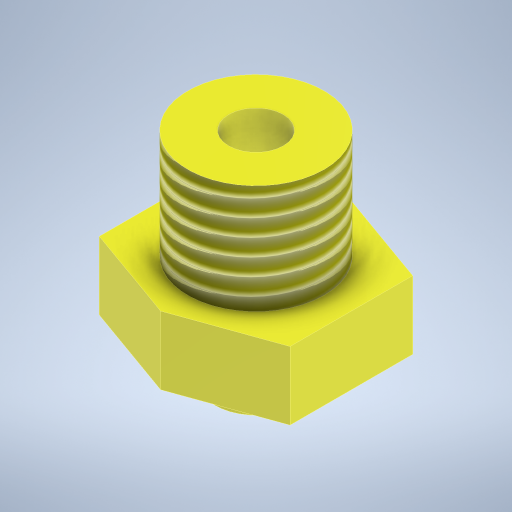
# Autodesk Inventor part: 1-HUDSON-8-30-TDR HAND PUMP BODY BOTTOM INLET
Saved by Autodesk Inventor 2024.2 (Build 282272000, 272)
## iProperties
Created: 2024-11-02
Part Number: 1-HUDSON-8-30-TDR HAND PUMP BODY BOTTOM INLET
Material: Genérico
Document SubType Name: Modeling
Designer: brene
Density: 1 g/cm^3
Appearance: Amarillo
Author: brene
Autodesk Inventor part; units mm, degrees
ref_plane "YZ Plane" through (0, 0, 0) normal (1, 0, 0) x (0, 1, 0)
ref_plane "XZ Plane" through (0, 0, 0) normal (0, 1, 0) x (-1, 0, 0)
ref_plane "XY Plane" through (0, 0, 0) normal (0, 0, 1) x (1, 0, 0)
sketch "Boceto1" plane through (0, 0, 0) normal (0, 0, 1) x (1, 0, 0)
  line L0 (0, 21.3006) -> (0, 0)
  line L1 (0, 15.4538) -> (5, 15.4538)
  line L2 (5, 15.4538) -> (5, 7.4538)
  line L3 (5, 7.4538) -> (0, 7.4538)
  line L4 (7, 7.4538) -> (5, 7.4538)
  line L5 (7, 7.4538) -> (7, 2.4538)
  line L6 (7, 2.4538) -> (0, 2.4538)
  line L7 (3, 2.4538) -> (3, 0.9538)
  line L8 (2, 15.4538) -> (2, -0.5462)
  line L9 (3, -0.5462) -> (2, -0.5462)
  line L10 (0, 0.6254) -> (0, -1.387)
  line L11 (3, -0.5462) -> (3, -0.5462)
  arc A0 (6, 2.4538) -> (3, -0.5462) centre (6, -0.5462) ccw
  line L12 (3, 0.9538) -> (3, -0.5462)
  point P0 (2, 2.4538)
  point P1 (2, 7.4538)
  dimension "d0" = 10
  dimension "d1" = 4
  dimension "d2" = 14
  dimension "d4" = 5
  dimension "d6" = 8
  dimension "d9" = 15.4538
  dimension "d10" = 13.8468
  dimension "d11" = 1.8283
  dimension "d12" = 3.8408
  dimension "d16" = 3
  dimension "d17" = 1
  dimension "d18" = 4
  dimension "d19" = 0.5462
  dimension "d20" = 6
  dimension "d21" = 1
  constraints: 26 end point, 8 point on line, 5 vertical, 3 perpendicular, 2 horizontal, 2 point on circle, 1 centre point, 1 collinear, 1 tangent
  measures "d0" diameter of L2 L0
  measures "d1" diameter of L8 L0
  measures "d2" diameter of L5 L0
  measures "d4" distance of L4.start L5.end
  measures "d6" distance of L1.end L2.end
  measures "d9" distance from line of L0.end L1
  measures "d10" distance from line of L0.start L4
  measures "d11" distance from line of L10.start L6
  measures "d12" distance from line of L10.end L6
  measures "d16" distance of L9.start L7.start
  measures "d17" distance of L9.start L8.end
  measures "d18" diameter of L8.end L10
  measures "d19" distance from line of L9 L0.end
  measures "d20" diameter of L7 L0
  measures "d21" distance of L5.end A0.start
revolve "Revolución1" add sketch "Boceto1" angle 360 about axis through (0, 21.3006, 0) along (0, -1, 0) contours L1 L2 L3 L8 | L3 L4 L5 L6 L8 | L6 L7 L12 L9 L8
revolve "Revolución2" add sketch "Boceto1" angle 360 about axis through (0, 0.6254, 0) along (0, -1, 0) contours L6 A0 L12 L7
sketch "Boceto2" plane through (0, 7.4538, 0) normal (0, 1, 0) x (1, 0, 0)
  line L0 (0, 11.3393) -> (0, -11.3393) construction
  line L1 (-23.3185, 0) -> (23.3185, 0) construction
  line L2 (7, 4.5) -> (7, -4.5)
  line L3 (-7, 4.5) -> (-7, -4.5)
  circle A0 centre (0, 0) radius 7 projected
  line L4 (-7, 4.5) -> (0, 7)
  line L5 (0, 7) -> (7, 4.5)
  line L6 (-7, -4.5) -> (0, -7)
  line L7 (7, -4.5) -> (0, -7)
  arc A1 (0, 7) -> (-4.4344, 5.4163) centre (0, 0) ccw
  arc A2 (4.4344, 5.4163) -> (0, 7) centre (0, 0) ccw
  arc A3 (0, -7) -> (4.4344, -5.4163) centre (0, 0) ccw
  arc A4 (-4.4344, -5.4163) -> (0, -7) centre (0, 0) ccw
  point P0 (7, 0)
  point P1 (-7, 0)
  point P2 (0, -7)
  point P3 (0, -7)
  point P4 (0, 7)
  point P5 (0, 7)
  point P6 (7, 0)
  point P7 (-7, 0)
  dimension "d24" = 9
  dimension "d26" = 9
  dimension "d27" = 7
  dimension "d28" = 7
  constraints: 16 end point, 12 point on circle, 8 point on line, 4 centre point, 4 concentric, 4 midpoint, 3 vertical, 2 tangent, 1 coincident, 1 horizontal, 1 parallel
  measures "d24" distance of L2.start L2.end
  measures "d26" distance of L3.start L3.end
  measures "d27" horizontal distance of point (0, 0) L3.start
  measures "d28" distance of point (0, 0) L4.end
extrude "Extrusión1" cut sketch "Boceto2" against normal through all contours A0 L7 | A0 L6
extrude "Extrusión2" cut sketch "Boceto2" against normal through all contours L5 A0 | L4 A0
extrude "Extrusión3" add sketch "Boceto2" against normal blind 5 contours L2 A0 L5 | L2 L7 A0 | A0 L3 L4 | L6 L3 A0
thread "Rosca1" size "M10x1.25" class "6g" standard "ANSI Metric M Profile" length 14
